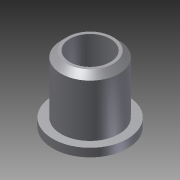
# Autodesk Inventor part: M20ANG1A2M201BR-bushing
Saved by Autodesk Inventor 2011 SP1 (Build 150282100, 282)
## iProperties
Created: 2013-12-24
Part Number: M20ANG1A2M201BR-bushing
Catalog Web Link: www.cadenas.de
Description: Angle Mount Miniature Toggles - Bushing-Series M - Miniature Toggles
Vendor: NKKSWITCHES
Document SubType Name: Modeling
Designer: PARTuser1
Manufacturer: NKKSWITCHES
Density: 1 g/cm^3
Category: PARTsolutions
Company: NKKSWITCHES
Title: M20ANG1A2M201BR-bushing
Author: Cadenas PARTsolutions
Comments: Series M - Miniature Toggles
PSOL_IDENT_0: {$CADENAS_DATA\23d-libs\nkkswitches\toggle\m\parts\m_ang_t_cover.prj},230 {VTYP=3D},{NB=M20ANG1A2M20
PSOL_IDENT_1: 1BR-bushing},{LINA=M20ANG1A2M201BR-bushing},{NN=Angle Mount Miniature Toggles - Bushing},{DATE=31.05
PSOL_IDENT_2: .2007 10:29:14},{GEOMDATE=31.05.2007 00:00:00},{VERSION=},{LINEID=10},{LINESUBID=-1},{WBVAR=PLS,BSHN
PSOL_IDENT_3: G}  {NB=M20ANG1A2M201BR-bushing},{LINA=M20ANG1A2M201BR-bushing},{KT=DUMMY},{PN=M20ANG1A2M201BR},{SRS
PSOL_IDENT_4: =M20},{PLS=1},{BSHNGALG='S1', 'S1 - .350\" (8.9mm) Threaded with Keyway','S2', 'S2 - .350\" (8.9mm)
PSOL_IDENT_5: Smooth with Keyway','A1', 'A1 - .280\" (7.1mm) Threaded with Keyway','A2', 'A2 - .280\" (7.1mm) Smoo
PSOL_IDENT_6: th with Keyway','L2', 'L2 - Smooth with Keyway for Lever Lock'},{BSHNG=A2},{WIDTH=0.512},{HEIGHT=0.3
PSOL_IDENT_7: 7},{LENGTH=0.311},{A=0},{TRMNLNOH=1},{DMAJ=0.244},{DMIN=0},{BSHNGDIA=0.315},{THRDL=0.285},{THRDL2=0.
PSOL_IDENT_8: 035},{PCDIA=0.256},{PC2=0.22},{PC3=0.024},{KEYPOS=0.098},{KEYW=0.031}
CNS_NN: Angle Mount Miniature Toggles - Bushing
CNS_NT: Series M - Miniature Toggles
CNS_NB: M20ANG1A2M201BR-bushing
CNS_NBSYN: $PN.-bushing
CNS_LINA: M20ANG1A2M201BR-bushing
CNS_PN: M20ANG1A2M201BR
CNS_SRS: M20
CNS_PLS: 1 - SPST/SPDT
CNS_BSHNGALG: 'S1', 'S1 - .350" (8.9mm) Threaded with Keyway','S2', 'S2 - .350" (8.9mm) Smooth with Keyway','A1', 'A1 - .280" (7.1mm) Threaded with Keyway','A2', 'A2 - .280" (7.1mm) Smooth with Keyway','L2', 'L2 - Smooth with Keyway for Lever Lock'
CNS_BSHNG: A2 - .280" (7.1mm) Smooth with Keyway
CNS_WIDTH: 0.512
CNS_HEIGHT: 0.370
CNS_LENGTH: 0.311
CNS_A: 0.000
CNS_TRMNLNOH: 1.000
CNS_DMAJ: 0.244
CNS_DMIN: 0.000
CNS_BSHNGDIA: 0.315
CNS_THRDL: 0.285
CNS_THRDL2: 0.035
CNS_PCDIA: 0.256
CNS_PC2: 0.220
CNS_PC3: 0.024
CNS_KEYPOS: 0.098
CNS_KEYW: 0.031
SUPPLIER: NKKSWITCHES
ARTICLENO: M20ANG1A2M201BR-bushing
BOMINFO: M20ANG1A2M201BR-bushing
CREATOR: CADENAS GmbH
Autodesk Inventor part; units mm, degrees
sketch "Sketch_1" plane through (0, 0, 0) normal (0, 0, 1) x (1, 0, 0)
  line L0 (-3.9497, 0) -> (3.9497, 0)
  arc A0 (3.9497, 0) -> (3.6957, 0.254) centre (3.6957, 0) ccw
  line L1 (3.6957, 0.254) -> (-3.6957, 0.254)
  arc A1 (-3.6957, 0.254) -> (-3.9497, 0) centre (-3.6957, 0) ccw
  constraints: 4 end point, 4 point on circle, 2 centre point
extrude "Extrusion1" add sketch "Sketch_1" along normal mid plane 13.0048
sketch "Sketch_7" plane through (0, 0, 0) normal (0, 0, 1) x (1, 0, 0)
  line L0 (0, 0.127) -> (0, 7.62)
  line L1 (0, 7.62) -> (2.479, 7.62)
  line L2 (2.479, 7.62) -> (3.0988, 7.0002)
  line L3 (3.0988, 7.0002) -> (3.0988, 1.397)
  line L4 (3.0988, 1.397) -> (4.0005, 1.397)
  line L5 (4.0005, 1.397) -> (4.0005, 0.508)
  line L6 (4.0005, 0.508) -> (3.2537, 0.508)
  line L7 (3.2537, 0.508) -> (3.2537, 0.127)
  line L8 (3.2537, 0.127) -> (0, 0.127)
  line L9 (0, 0.127) -> (0, 7.62)
  constraints: 20 end point
revolve "Revolution1" add sketch "Sketch_7" angle 360 about axis through (0, 0.127, 0) along (0, -1, 0)
sketch "Sketch_8" plane through (0, 0.254, 0) normal (0, 1, 0) x (1, 0, 0)
  line L0 (-0.3937, 2.4892) -> (0.3937, 2.4892)
  line L1 (0.3937, 2.4892) -> (0.3937, 10.4902)
  line L2 (0.3937, 10.4902) -> (-0.3937, 10.4902)
  line L3 (-0.3937, 10.4902) -> (-0.3937, 2.4892)
  constraints: 8 end point
extrude "Extrusion2" cut sketch "Sketch_8" along normal blind 7.9629
sketch "Sketch4" plane through (-3.9497, 0, 6.5024) normal (0, -1, 0) x (1, 0, 0)
  point P0 (3.9497, -6.5024)
hole "Drilling 1" at (0, 0, 0) direction (0, 1, 0) diameter 4.3383 depth 7.874
sketch "Sketch_2" plane through (0, 0, 0) normal (0, 0, 1) x (1, 0, 0)
  line L0 (-3.9497, 0.254) -> (-3.9497, 0)
  line L1 (-3.9497, 0) -> (3.9497, 0)
  line L2 (3.9497, 0) -> (3.9497, 0.254)
  line L3 (3.9497, 0.254) -> (-3.9497, 0.254)
  constraints: 8 end point
extrude "Extrusion3" cut sketch "Sketch_2" along normal mid plane 13.0048
ref_plane "1_XY" through (0, 5.7912, 0) normal (0, 1, 0) x (1, 0, 0)
ref_plane "1_YZ" through (0, 5.7912, 0) normal (1, 0, 0) x (0, 0, -1)
ref_plane "1_ZX" through (0, 5.7912, 0) normal (0, 0, -1) x (0, 1, 0)
ref_plane "2_XY" through (0, 4.3434, 0) normal (0, 1, 0) x (1, 0, 0)
ref_plane "2_YZ" through (0, 4.3434, 0) normal (1, 0, 0) x (0, 0, -1)
ref_plane "2_ZX" through (0, 4.3434, 0) normal (0, 0, -1) x (0, 1, 0)
ref_plane "3_XY" through (0, 2.8956, 0) normal (0, 1, 0) x (1, 0, 0)
ref_plane "3_YZ" through (0, 2.8956, 0) normal (1, 0, 0) x (0, 0, -1)
ref_plane "3_ZX" through (0, 2.8956, 0) normal (0, 0, -1) x (0, 1, 0)
ref_plane "4_XY" through (0, 1.8097, 0) normal (0, 1, 0) x (1, 0, 0)
ref_plane "4_YZ" through (0, 1.8097, 0) normal (1, 0, 0) x (0, 0, -1)
ref_plane "4_ZX" through (0, 1.8097, 0) normal (0, 0, -1) x (0, 1, 0)
ref_plane "to_base_XY" through (0, 0, 0) normal (0, 1, 0) x (1, 0, 0)
ref_plane "to_base_YZ" through (0, 0, 0) normal (1, 0, 0) x (0, 0, -1)
ref_plane "to_base_ZX" through (0, 0, 0) normal (0, 0, -1) x (0, 1, 0)
body "Solid1"
